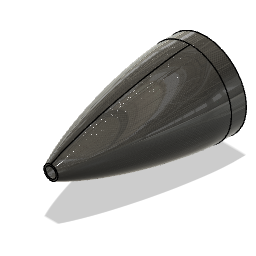
Baugruppe Rakete v7 (Autodesk Fusion 360 archive; units mm, degrees)
design "Nosecone carbon 25.10.2024"
Autodesk Fusion 360 part; units mm, degrees
sketch "Skizze1" plane through (0, 0, 0) normal (1, 0, 0) x (0, 0, -1)
  line L0 (-260, 23.37) -> (-280, 14.04)
  line L1 (-280, 14.04) -> (-290, 8.39)
  line L2 (-260, 23.37) -> (-230, 34.95)
  line L3 (-230, 34.95) -> (-200, 44.83)
  line L4 (-200, 44.83) -> (-160, 56.15)
  line L5 (-160, 56.15) -> (-130, 63.46)
  line L6 (-300, 0) -> (-298, 2.52)
  line L7 (-298, 2.52) -> (-295, 5)
  line L8 (-295, 5) -> (-290, 8.39)
  line L9 (-130, 63.46) -> (-90, 71.77)
  line L10 (-90, 71.77) -> (-40, 79.64)
  line L11 (-40, 79.64) -> (-20, 81.8)
  line L12 (-20, 81.8) -> (0, 83)
  line L13 (0, 83) -> (30, 83)
  line L14 (0, 83) -> (30, 83)
  spline S0 degree 5 poles (0, 83) (-0.9322, 82.957) (-2.773, 82.87) (-5.4634, 82.7359) (-8.9088, 82.5503) (-12.9885, 82.3057) (-16.8689, 82.0449) (-20.6061, 81.7609) (-24.2951, 81.4421) (-28.0746, 81.0712) (-32.1002, 80.6288) (-36.519, 80.0963) (-41.4457, 79.4587) (-46.9344, 78.7077) (-52.9648, 77.8437) (-59.4623, 76.8738) (-66.3117, 75.8102) (-73.373, 74.6692) (-80.4964, 73.4695) (-87.5381, 72.2308) (-94.3743, 70.9725) (-100.9194, 69.7121) (-107.1274, 68.4642) (-112.986, 67.24) (-118.512, 66.0461) (-123.7467, 64.8844) (-128.7513, 63.7504) (-133.602, 62.6333) (-138.3859, 61.5146) (-143.1932, 60.3702) (-148.1077, 59.1751) (-153.1987, 57.9063) (-158.5112, 56.5469) (-164.0583, 55.0892) (-169.8093, 53.5395) (-175.6984, 51.9155) (-181.6391, 50.2416) (-187.5373, 48.5452) (-193.3043, 46.8522) (-198.8707, 45.1828) (-204.1986, 43.5481) (-209.2975, 41.9444) (-214.2149, 40.3564) (-219.0198, 38.7624) (-223.7881, 37.138) (-228.5873, 35.4614) (-233.4626, 33.7172) (-238.4192, 31.9016) (-243.426, 30.0219) (-248.4287, 28.0928) (-253.3595, 26.1341) (-258.1484, 24.1679) (-262.7328, 22.2157) (-267.0706, 20.2957) (-271.1406, 18.4217) (-274.9346, 16.6044) (-278.4519, 14.8519) (-281.6937, 13.1703) (-284.6552, 11.5645) (-287.3272, 10.0386) (-289.706, 8.5968) (-291.8012, 7.243) (-293.6459, 5.983) (-295.2821, 4.8116) (-296.74, 3.695) (-298.0233, 2.5618) (-298.9053, 1.5894) (-299.4846, 0.813) (-299.8343, 0.2745) (-300, 0) knots 0 0 0 0 0 0 0.01538462 0.03076923 0.04615385 0.06153846 0.07692308 0.09230769 0.10769231 0.12307692 0.13846154 0.15384615 0.16923077 0.18461538 0.2 0.21538462 0.23076923 0.24615385 0.26153846 0.27692308 0.29230769 0.30769231 0.32307692 0.33846154 0.35384615 0.36923077 0.38461538 0.4 0.41538462 0.43076923 0.44615385 0.46153846 0.47692308 0.49230769 0.50769231 0.52307692 0.53846154 0.55384615 0.56923077 0.58461538 0.6 0.61538462 0.63076923 0.64615385 0.66153846 0.67692308 0.69230769 0.70769231 0.72307692 0.73846154 0.75384615 0.76923077 0.78461538 0.8 0.81538462 0.83076923 0.84615385 0.86153846 0.87692308 0.89230769 0.90769231 0.92307692 0.93846154 0.95384615 0.96923077 0.98461538 1 1 1 1 1 1
  line L15 (0.1381, 80.0032) -> (30, 80.0032)
  line L16 (30, 80.0032) -> (30, 83)
  spline S1 degree 3 poles (0.1381, 80.0032) (-5.3956, 79.7482) (-10.3945, 79.4727) (-14.9862, 79.1606) (-18.9745, 78.8896) (-22.6391, 78.5928) (-26.579, 78.197) (-30.2006, 77.8332) (-34.1163, 77.3785) (-38.8034, 76.7706) (-43.3782, 76.1772) (-48.6992, 75.4362) (-54.6181, 74.5583) (-62.8597, 73.336) (-72.212, 71.8504) (-81.2998, 70.2728) (-88.6532, 68.9963) (-95.784, 67.6657) (-102.3101, 66.3651) (-109.346, 64.9629) (-115.6909, 63.5997) (-121.531, 62.2994) (-130.6599, 60.2669) (-138.6135, 58.4165) (-147.4068, 56.2505) (-152.4678, 55.0039) (-157.8323, 53.634) (-163.547, 52.1114) (-171.5204, 49.9869) (-180.1377, 47.5749) (-188.3041, 45.1883) (-193.9882, 43.5271) (-199.4138, 41.8911) (-204.4798, 40.3083) (-210.9231, 38.295) (-216.8267, 36.3556) (-222.7977, 34.2958) (-227.6528, 32.6209) (-232.5948, 30.8535) (-237.6449, 28.9777) (-245.8863, 25.9164) (-254.3169, 22.5835) (-261.6486, 19.3972) (-270.0166, 15.7604) (-276.9857, 12.3321) (-282.3719, 9.3784) (-285.7999, 7.4985) (-288.5366, 5.8129) (-290.7419, 4.3239) (-292.7166, 2.9906) (-294.3202, 1.8334) (-295.4633, 0.7925) (-296.31, 0.0214) (-296.9311, -0.7211) (-297.4317, -1.5504) knots 0 0 0 0 0.054964 0.054964 0.054964 0.102705 0.102705 0.102705 0.14659 0.14659 0.14659 0.189423 0.189423 0.189423 0.249066 0.249066 0.249066 0.297325 0.297325 0.297325 0.349355 0.349355 0.349355 0.430685 0.430685 0.430685 0.477496 0.477496 0.477496 0.542809 0.542809 0.542809 0.58827 0.58827 0.58827 0.646091 0.646091 0.646091 0.693105 0.693105 0.693105 0.769829 0.769829 0.769829 0.857397 0.857397 0.857397 0.91313 0.91313 0.91313 0.963033 0.963033 0.963033 1 1 1 1
  line L17 (-300, 0) -> (-296.2633, 0)
  line L18 (-280, 14.04) -> (-280, 10.6551)
  dimension "d1" = 10
  dimension "d2" = 8.39
  dimension "d4" = 20
  dimension "d5" = 40
  dimension "d6" = 70
  dimension "d7" = 300
  dimension "d8" = 100
  dimension "d9" = 140
  dimension "d10" = 170
  dimension "d11" = 14.04
  dimension "d12" = 2
  dimension "d13" = 5
  dimension "d14" = 2.52
  dimension "d15" = 5
  dimension "d16" = 23.37
  dimension "d17" = 34.95
  dimension "d18" = 44.83
  dimension "d19" = 56.15
  dimension "d20" = 63.46
  dimension "d21" = 210
  dimension "d22" = 260
  dimension "d23" = 71.77
  dimension "d24" = 79.64
  dimension "d25" = 83
  dimension "d26" = 280
  dimension "d27" = 81.8
  dimension "d28" = 30
  dimension "d30" = -3
  constraint horizontal origin L6.start
  constraint vertical origin L12.end
  constraint horizontal L13
  constraint parallel L14 L15
  constraint vertical L16
  constraint coincident L15.start S1.start
  constraint coincident S1 L17.end
  constraint horizontal L17
  constraint coincident L0.end L1.start
  constraint coincident S1 L18.end
  constraint vertical L18
  measures "d1" horizontal distance of L1.end L6.start
  measures "d2" vertical distance of L1.end L6.start
  measures "d4" horizontal distance of L0.end L6.start
  measures "d5" horizontal distance of L0.start L6.start
  measures "d6" horizontal distance of L6.start L2.end
  measures "d7" distance of origin L6.start
  measures "d8" horizontal distance of L3.end L6.start
  measures "d9" horizontal distance of L6.start L4.end
  measures "d10" horizontal distance of L6.start L5.end
  measures "d11" vertical distance of L0.end L6.start
  measures "d12" horizontal distance of L6.start L6.end
  measures "d13" horizontal distance of L6.start L7.end
  measures "d14" vertical distance of L6.start L6.end
  measures "d15" vertical distance of L6.start L7.end
  measures "d16" vertical distance of L0.start L6.start
  measures "d17" vertical distance of L6.start L2.end
  measures "d18" vertical distance of L3.end L6.start
  measures "d19" vertical distance of L6.start L4.end
  measures "d20" vertical distance of L6.start L5.end
  measures "d21" horizontal distance of L6.start L9.end
  measures "d22" horizontal distance of L6.start L10.end
  measures "d23" vertical distance of L6.start L9.end
  measures "d24" vertical distance of L6.start L10.end
  measures "d25" vertical distance of L6.start L12.end
  measures "d26" horizontal distance of L6.start L11.end
  measures "d27" vertical distance of L6.start L11.end
  measures "d28" distance of L12.end L13.end
revolve "Drehen1" add sketch "Skizze1" angle 360 about axis through (0, 0, 1.75) along (0, 0, 1) contours L0 L2 L3 L4 L5 L9 L10 L11 L12 L13 L14 L15 L16 S1 L18 | L2 S0 | L0 S0 | L3 S0 | L4 S0 | L5 S0 | L9 S0 | L10 S0 | L12 S0 | L11 S0
fillet "Abrundung1" radius 2 1 edges at (-74.5892, 28.9304, -30)

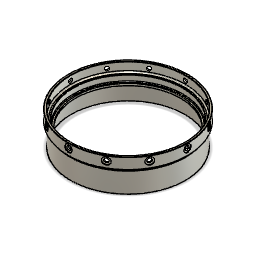
design "Connection-Ring-female-21.10.2024"
Autodesk Fusion 360 part; units mm, degrees
sketch "Skizze1" plane through (0, 0, 0) normal (0, 0, 1) x (1, 0, 0)
  line L0 (-83, 47) -> (-83, 30)
  line L1 (-83, 30) -> (-80, 30)
  line L2 (-80, 30) -> (-80, 0)
  line L3 (-73, 22.5) -> (-73, 25.5)
  line L4 (-73, 25.5) -> (-76, 25.5)
  line L5 (-76, 25.5) -> (-76, 34)
  line L6 (-76, 34) -> (-80, 34)
  line L7 (-80, 34) -> (-80, 47)
  line L8 (-80, 47) -> (-83, 47)
  line L9 (-80, 0) -> (-79, 0)
  line L10 (-76.75, 22.5) -> (-73, 22.5)
  line L11 (-76.75, 22.5) -> (-79, 0)
  line L12 (-76, 30) -> (-76.75, 22.5)
  dimension "d2" = 3
  dimension "d6" = 13
  dimension "d7" = 80
  dimension "d8" = 3
  dimension "d9" = 4
  dimension "d10" = 3
  dimension "d21" = 4
  dimension "d22" = 8.5
  dimension "d23" = 3
  dimension "d24" = 30
  dimension "d25" = 1
  constraint vertical L0
  constraint perpendicular L0 L1
  constraint perpendicular L1 L2
  constraint perpendicular L2 L4
  constraint perpendicular L5 L6
  constraint perpendicular L6 L7
  constraint perpendicular L0 L8
  constraint perpendicular L2 L9
  constraint horizontal origin L2.end
  constraint coincident L5 L12.start
  constraint collinear L11 L12
  constraint horizontal L1.end L12.start
  measures "d2" distance of L3 L5
  measures "d6" distance of L6 L8
  measures "d7" distance of origin L2
  measures "d8" distance of L0 L7
  measures "d9" distance of L2 L5
  measures "d10" distance of L0 L2
  measures "d21" distance of L1 L6
  measures "d22" distance of L4 L6
  measures "d23" distance of L4 L10
  measures "d24" distance of L1 L9
  measures "d25" distance of L2.end L9.end
revolve "Drehen1" add sketch "Skizze1" angle 360 about axis through (0, 1.75, 0) along (0, 1, 0)
fillet "Abrundung1" radius 2 1 edges at (-77.3832, 30, 30.0141)
fillet "Abrundung2" radius 2 1 edges at (-74.5862, 30, 28.9292)
fillet "Abrundung3" radius 2 1 edges at (-74.5862, 34, 28.9292)
chamfer "Fase3" distance 1 angle 45 1 edges at (-70.8569, 25.5, 27.4828)
ref_plane "Arbeitsebene1" through (83, 38.5, 0) normal (1, 0, 0) x (0, 0, -1)
sketch "Skizze4" plane through (83, 0, 0) normal (1, 0, 0) x (0, 0, -1)
  line L0 (-82.5, 47) -> (82.5, 47)
  point P0 (0, 40.5)
  dimension "d34" = 6.5
  constraint vertical origin P0
  measures "d34" distance of P0 L0
hole "Bohrung2" at (83, 40.5, 0) direction (-1, 0, 0) diameter 5.5 depth 16 tip angle 118 counterbore diameter 10 counterbore depth 1
pattern_circular "C-Anordnung1" count 12 over 360 about axis through (0, 1.75, 0) along (0, 1, 0) of "Bohrung2"
chamfer "Fase4" distance 0.4 angle 45 7 edges at (-74.5862, 47, 28.9292) (-70.8569, 34, 27.4828) (-74.5862, 0, 28.9292) (-73.6539, 0, 28.5676) (-71.5561, 22.5, 27.754) (-68.0599, 22.5, 26.3979) (-77.3832, 47, 30.0141)
equation "d7 = ( 160 / 2 ) * 1 mm"
equation "d22 = 15 mm - d6 / 2"

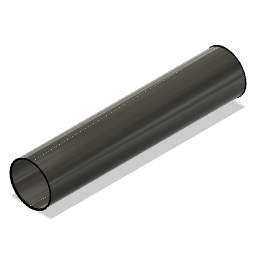
design "Computer/Nutzlastsektion 800"
Autodesk Fusion 360 part; units mm, degrees
sketch "Skizze1" plane through (0, 0, 0) normal (0, 0, 1) x (1, 0, 0)
  circle A0 centre (0, 0) radius 80
  circle A1 centre (0, 0) radius 83
  dimension "d1" = 166
  dimension "d2" = 160
  constraint coincident A0.centre A1.centre
  constraint concentric A0 A1
  measures "d1" diameter of A1
  measures "d2" diameter of A0
extrude "Extrusion1" add sketch "Skizze1" along normal blind 800
fillet "Abrundung1" radius 2 2 edges at (-74.5862, 28.9292, 800) (-74.5862, 28.9292, 0)

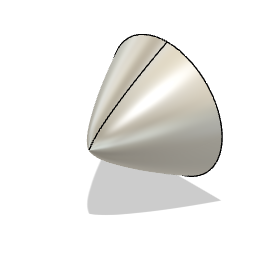
design "Nasenspitze"
Autodesk Fusion 360 part; units mm, degrees
sketch "Skizze1" plane through (0, 0, 0) normal (1, 0, 0) x (0, 0, -1)
  line L0 (-18, 2.52) -> (-15, 5)
  line L1 (-15, 5) -> (-10, 8.39)
  line L2 (0, 14.04) -> (-10, 8.39)
  line L3 (-20, 0) -> (-18, 2.52)
  spline S0 degree 5 poles (0, 14.04) (-0.347, 13.8595) (-1.0331, 13.5009) (-2.0382, 12.9697) (-3.3302, 12.2751) (-4.8637, 11.4299) (-6.3143, 10.6085) (-7.6808, 9.8116) (-8.9624, 9.0402) (-10.1599, 8.2952) (-11.2757, 7.5774) (-12.3148, 6.8876) (-13.2837, 6.2257) (-14.189, 5.5902) (-15.0369, 4.9781) (-15.8322, 4.3839) (-16.5772, 3.7988) (-17.2729, 3.2129) (-17.9192, 2.6164) (-18.5158, 2.001) (-19.0631, 1.362) (-19.4619, 0.8303) (-19.7393, 0.4197) (-19.9147, 0.1408) (-20, 0) knots 0 0 0 0 0 0 0.05 0.1 0.15 0.2 0.25 0.3 0.35 0.4 0.45 0.5 0.55 0.6 0.65 0.7 0.75 0.8 0.85 0.9 0.95 1 1 1 1 1 1
  line L4 (-20, 0) -> (-15, 0)
  line L5 (0, 10) -> (0, 14.04)
  line L6 (0, 10) -> (-14.017, 1.7221)
  arc A0 (-14.017, 1.7221) -> (-15, 0) centre (-13, 0) ccw
  point P0 (-297.4317, -1.5504)
  dimension "d1" = 10
  dimension "d2" = 8.39
  dimension "d3" = 20
  dimension "d4" = 14.04
  dimension "d5" = 2
  dimension "d6" = 5
  dimension "d7" = 2.52
  dimension "d8" = 5
  dimension "d9" = 15
  dimension "d10" = 10
  dimension "d11" = 2
  constraint vertical origin L2.start
  constraint horizontal origin L3.start
  constraint horizontal L4
  constraint vertical L5
  constraint tangent L6 A0
  constraint horizontal origin A0.centre
  measures "d1" horizontal distance of L3.start L1.end
  measures "d2" vertical distance of L3.start L1.end
  measures "d3" horizontal distance of L3.start L2.start
  measures "d4" vertical distance of L3.start L2.start
  measures "d5" horizontal distance of L3.start L0.start
  measures "d6" horizontal distance of L3.start L0.end
  measures "d7" vertical distance of L3.start L0.start
  measures "d8" vertical distance of L3.start L0.end
  measures "d9" distance of origin L4.end
  measures "d10" distance of origin L5.start
  measures "d11" radius of A0
revolve "Drehen1" add sketch "Skizze1" angle 360 about axis through (0, 0, 1.75) along (0, 0, 1)

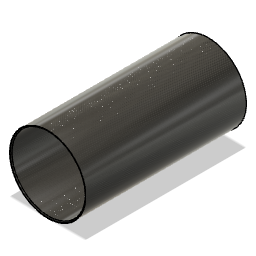
design "Antriebssektion 2 350"
Autodesk Fusion 360 part; units mm, degrees
sketch "Skizze1" plane through (0, 0, 0) normal (0, 0, 1) x (1, 0, 0)
  circle A0 centre (0, 0) radius 83
  circle A1 centre (0, 0) radius 80
  dimension "d1" = 160
  dimension "d2" = 166
  constraint coincident A0.centre A1.centre
  measures "d1" diameter of A1
  measures "d2" diameter of A0
extrude "Extrusion1" add sketch "Skizze1" along normal blind 350
fillet "Abrundung1" radius 2 2 edges at (-74.5862, 28.9292, 350) (-74.5862, 28.9292, 0)

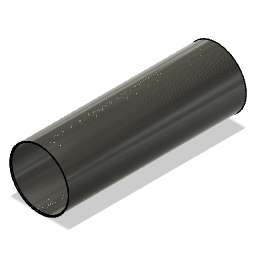
design "Antriebssektion 1 500"
Autodesk Fusion 360 part; units mm, degrees
sketch "Skizze1" plane through (0, 0, 0) normal (0, 0, 1) x (1, 0, 0)
  circle A0 centre (0, 0) radius 83
  circle A1 centre (0, 0) radius 80
  dimension "d1" = 166
  dimension "d2" = 160
  constraint coincident A0.centre A1.centre
  constraint concentric A0 A1
  measures "d1" diameter of A0
  measures "d2" diameter of A1
extrude "Extrusion1" add sketch "Skizze1" along normal blind 500
fillet "Abrundung1" radius 2 2 edges at (-74.5862, 28.9292, 500) (-74.5862, 28.9292, 0)

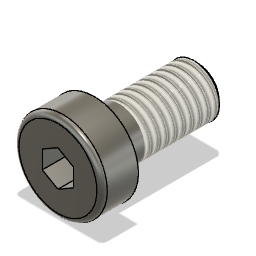
design "Innensechskantschraube DIN 7984 - M5 x 10 Stahl 8.8 Einfach"
description: Innensechskantschraube DIN 7984 - M5 x 10
Autodesk Fusion 360 part; units mm, degrees
sketch "Sketch1" plane through (0, 0, 0) normal (0, 1, 0) x (1, 0, 0)
  line L0 (-2.5, 0) -> (-2.5, 10)
  line L1 (-2.5, 10) -> (0, 10)
  line L2 (0, 10) -> (0, -3.5)
  line L3 (-2.5, 0) -> (-4.25, 0)
  line L4 (-4.25, 0) -> (-4.25, -3.5)
  line L5 (-4.25, -3.5) -> (0, -3.5)
  dimension "d9" = 5
  dimension "d66" = 8.5
  dimension "d68" = 10
  dimension "d79" = 3.5
  constraint perpendicular L0 L1
  constraint collinear origin L1.end L2.end
  constraint perpendicular L0 L3
  constraint coincident origin L3
  constraint vertical L0
  constraint vertical L2
  constraint parallel L2 L4
  constraint coincident L2 L5.end
  constraint perpendicular L2 L5
  measures "d68" distance of origin L1.end
  measures "d79" distance of L3.end L4.end
revolve "Revolve1" add sketch "Sketch1" angle 360 about axis through (0, 0, -10) along (0, 0, 1)
ref_plane "WorkPlane1" through (0, 0, 3.5) normal (0, 0, 1) x (1, 0, 0)
sketch "Sketch6" plane through (0, 0, 3.5) normal (0, 0, 1) x (1, 0, 0)
  line L0 (-1.5, 0) -> (1.5, 0) construction
  line L1 (0, 0) -> (-1.5, 0.866)
  line L2 (-1.5, -0.866) -> (-1.5, 0.866)
  line L3 (-1.5, -0.866) -> (0, 0)
  dimension "d72" = 3
  dimension "d100" = 150
  constraint horizontal L0
  constraint midpoint L1.start L0
  constraint coincident L1.start L3.end
  constraint perpendicular L0 L2
  constraint midpoint L0.start L2
  constraint coincident L1.end L2.end
  measures "d72" distance of L0.start L0.end
  measures "d100" angle of L0 L1
extrude "Extrude1" cut sketch "Sketch6" against normal blind 2.7
pattern_circular "C-Pattern1" count 6 over 360 about axis through (0, 0, 1.75) along (0, 0, 1) of "Extrude1"
extrude "Extrude2" cut 1 faces at (0, -0.5774, 0.8) along direction (0, 0, -1) blind 2.7 draft -85
thread "Thread2" "ISO Metric profile 5.0 M5x0.8 6g" major diameter 4.901 minor diameter 3.9895 pitch 0.8 angle 60 resizes the face on face at (-2.4876, 0.2489, -3.3333) from (0, 0, -2.4) to (0, 0, -10)
fillet "Fillet4" radius 0.5 1 edges at (-3.9624, 1.5369, 3.5)
sketch "Sketch7" plane through (0, 0, 0) normal (0, 1, 0) x (1, 0, 0)
  line L0 (-2.55, 10) -> (-2.55, 9.5092)
  line L1 (-2.55, 9.5092) -> (-2.0092, 10)
  line L2 (0, 10) -> (0, -3.5)
  line L3 (-2.55, 10) -> (0, 10)
  dimension "d92" = 0.4908
  dimension "d98" = 2.0092
  dimension "d99" = 2.55
  constraint coincident L2.start L3.end
  constraint perpendicular L2 L3
  constraint coincident L1.end L3
  constraint perpendicular L0 L3
  measures "d92" vertical distance of L0.end L1.end
  measures "d98" horizontal distance of origin L1.end
  measures "d99" distance of origin L0
revolve "Revolve3" cut sketch "Sketch7" angle 360 about axis through (0, 0, 1.75) along (0, 0, 1)
equation "d9 = adsk_nomdia"
equation "adsk_nomlen = 10.00 mm"
equation "adsk_headh = 3.50 mm"
equation "adsk_headdia = 8.50 mm"
equation "adsk_nomdia = 5.00 mm"
equation "adsk_philwidth = 3.00 mm"
equation "d31 = -adsk_phildepth"
equation "adsk_phildepth = 2.70 mm"
equation "d66 = adsk_headdia"
equation "d68 = adsk_nomlen"
equation "d71 = adsk_headh"
equation "d72 = adsk_philwidth"
equation "d76 = -adsk_phildepth"
equation "d79 = adsk_headh"
equation "adsk_thrlen = 7.60 mm"
equation "d84 = adsk_thrlen"
equation "d86 = adsk_nomdia * 0.1"
equation "d92 = adsk_startlen"
equation "adsk_startlen = 0.49076 mm"
equation "adsk_endpointdia = 4.01848 mm"
equation "d98 = adsk_endpointdia / 2"
equation "d99 = adsk_nomdia * 0.51"

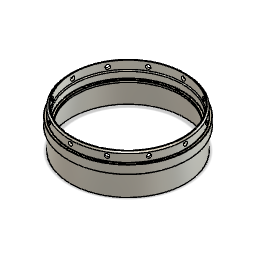
design "Connection-Ring-male-21.10.2024"
Autodesk Fusion 360 part; units mm, degrees
sketch "Skizze1" plane through (0, 0, 0) normal (0, 0, 1) x (1, 0, 0)
  line L0 (-80, 0) -> (-80, 30)
  line L1 (-80, 30) -> (-83, 30)
  line L2 (-83, 30) -> (-83, 42)
  line L3 (-83, 42) -> (-79.95, 42)
  line L4 (-79.95, 42) -> (-79.95, 53)
  line L5 (-77.95, 55) -> (-76.95, 55)
  line L6 (-76.95, 55) -> (-76.95, 42)
  line L7 (-76, 33.5) -> (-73, 33.5)
  line L8 (-73, 30.5) -> (-73, 33.5)
  line L9 (-77.95, 55) -> (-79.95, 53)
  line L10 (-80, 0) -> (-79, 0)
  line L11 (-73, 30.5) -> (-75.95, 30.5)
  line L12 (-75.95, 30.5) -> (-79, 0)
  line L13 (-76, 30) -> (-75.95, 30.5)
  line L14 (-76.95, 42) -> (-76, 42)
  line L15 (-76, 42) -> (-76, 33.5)
  dimension "d1" = 3
  dimension "d2" = 80
  dimension "d5" = 3
  dimension "d7" = 3.05
  dimension "d9" = 2
  dimension "d10" = 3
  dimension "d13" = 1
  dimension "d14" = 30
  dimension "d16" = 2
  dimension "d17" = 4
  dimension "d18" = 8.5
  dimension "d19" = 13
  dimension "d20" = 12
  dimension "d25" = 3
  constraint perpendicular L0 L1
  constraint perpendicular L1 L2
  constraint perpendicular L2 L3
  constraint perpendicular L3 L4
  constraint perpendicular L4 L5
  constraint perpendicular L3 L6
  constraint perpendicular L4 L7
  constraint perpendicular L7 L8
  constraint perpendicular L0 L10
  constraint vertical L8
  constraint perpendicular L8 L11
  constraint horizontal origin L0.start
  constraint collinear L12 L13
  constraint horizontal L0.end L13.start
  constraint perpendicular L6 L14
  constraint perpendicular L14 L15
  constraint vertical L7.start L13.start
  constraint collinear L3 L14
  measures "d1" distance of L7.end L8.start
  measures "d2" distance of origin L0
  measures "d5" distance of L4 L6
  measures "d7" distance of L2 L4
  measures "d9" distance of L4 L5.start
  measures "d10" distance of L0 L2
  measures "d13" distance of L0.start L10.end
  measures "d14" distance of L1 L10
  measures "d16" distance of L5 L4.end
  measures "d17" distance of L0.end L13.start
  measures "d18" distance of L3 L7
  measures "d19" distance of L3 L5
  measures "d20" distance of L1 L3
  measures "d25" distance of L8 L15
revolve "Drehen1" add sketch "Skizze1" angle 360 about axis through (0, 1.75, 0) along (0, 1, 0)
fillet "Abrundung1" radius 2 1 edges at (-71.7426, 42, 27.8263)
ref_plane "Arbeitsebene1" through (79.95, 47.5, 0) normal (1, 0, 0) x (0, 0, -1)
sketch "Skizze2" plane through (79.95, 0, 0) normal (1, 0, 0) x (0, 0, -1)
  line L0 (77.95, 55) -> (-77.95, 55)
  point P0 (0, 48.5)
  dimension "d27" = 6.5
  constraint vertical origin P0
  measures "d27" distance of P0 L0
hole "Bohrung1" at (79.95, 48.5, 0) direction (-1, 0, 0) diameter 5.5 depth 16 tip angle 118
pattern_circular "C-Anordnung1" count 12 over 360 about axis through (0, 1.75, 0) along (0, 1, 0) of "Bohrung1"
chamfer "Fase1" distance 0.4 angle 45 9 edges at (-77.3832, 42, 30.0141) (-77.3832, 30, 30.0141) (-73.6539, 0, 28.5676) (-70.8103, 30.5, 27.4647) (-68.0599, 30.5, 26.3979) (-70.8569, 33.5, 27.4828) (-74.5396, 42, 28.9112) (-74.5862, 0, 28.9292) (-68.0599, 33.5, 26.3979)
fillet "Abrundung2" radius 2 1 edges at (-74.5862, 30, 28.9292)
equation "d2 = ( 160 / 2 ) * 1 mm"
equation "d18 = 15 mm - d19 / 2"

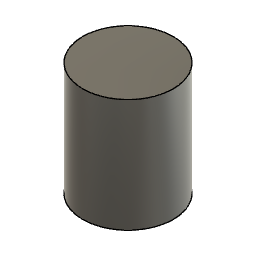
design "Bolzen"
Autodesk Fusion 360 part; units mm, degrees
sketch "Skizze1" plane through (0, 0, 0) normal (0, 1, 0) x (1, 0, 0)
  circle A0 centre (0, 0) radius 2
  dimension "d1" = 4
  constraint coincident A0.centre origin
  measures "d1" diameter of A0
extrude "Extrusion1" add sketch "Skizze1" along normal blind 5

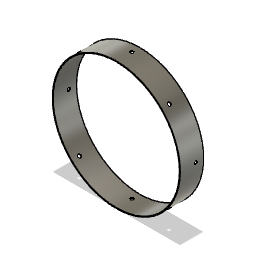
design "Kupplungsring Verbinder 25.10.2024"
Autodesk Fusion 360 part; units mm, degrees
sketch "Skizze2" plane through (0, 0, 0) normal (0, 0, 1) x (1, 0, 0)
  circle A0 centre (0, 0) radius 82
  circle A1 centre (0, 0) radius 81
  dimension "d1" = 164
  dimension "d2" = 162
  constraint coincident A0.centre A1.centre
  constraint concentric A0 A1
  measures "d1" diameter of A0
  measures "d2" diameter of A1
extrude "Extrusion1" add sketch "Skizze2" along normal blind 30
ref_plane "Arbeitsebene1" through (0, 82, 15) normal (0, 1, 0) x (-1, 0, 0)
sketch "Skizze3" plane through (0, 82, 0) normal (0, 1, 0) x (1, 0, 0)
  point P0 (0, -10)
  dimension "d6" = 10
  constraint vertical origin P0
  measures "d6" distance of origin P0
ref_plane "Arbeitsebene2" through (-57.9828, 57.9828, 15) normal (-0.707107, 0.707107, 0) x (-0.707107, -0.707107, 0)
sketch "Skizze4" plane through (-57.9828, 57.9828, 0) normal (-0.707107, 0.707107, 0) x (-0.707107, -0.707107, 0)
  line L0 (82, 30) -> (-82, 30)
  point P0 (0, 20)
  dimension "d8" = 10
  constraint vertical origin P0
  measures "d8" distance of P0 L0
hole "Bohrung1" at (0, 82, 10) direction (0, -1, 0) diameter 4 depth 35 tip angle 118
hole "Bohrung2" at (-57.9828, 57.9828, 20) direction (0.707107, -0.707107, 0) diameter 4 depth 35 tip angle 118
pattern_circular "C-Anordnung1" count 4 over 360 about axis through (0, 0, 1.75) along (0, 0, 1) of "Bohrung1", "Bohrung2"

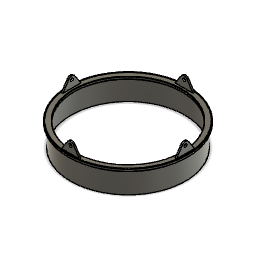
design "Kupplungsring 25.10.2024"
Autodesk Fusion 360 part; units mm, degrees
sketch "Skizze1" plane through (0, 0, 0) normal (0, 0, 1) x (1, 0, 0)
  line L0 (-80, 0) -> (-79, 0)
  line L1 (-79, 0) -> (-77, 30)
  line L2 (-77, 30) -> (-75, 30)
  line L3 (-75, 30) -> (-75, 33)
  line L4 (-80, 30) -> (-80, 0)
  line L5 (-80, 30) -> (-83, 30)
  line L6 (-83, 30) -> (-83, 35)
  line L7 (-82, 33) -> (-75, 33)
  line L8 (-83, 35) -> (-83, 33.5)
  line L9 (-83, 33.5) -> (-82, 33.5)
  line L10 (-82, 33.5) -> (-82, 33)
  dimension "d1" = 80
  dimension "d2" = 1
  dimension "d3" = 3
  dimension "d4" = 30
  dimension "d5" = 8
  dimension "d6" = 3
  dimension "d7" = 3
  dimension "d8" = 1
  dimension "d9" = 0.5
  constraint horizontal L0
  constraint parallel L0 L2
  constraint perpendicular L2 L3
  constraint perpendicular L0 L4
  constraint horizontal origin L0.end
  constraint perpendicular L4 L5
  constraint perpendicular L5 L6
  constraint horizontal L7
  constraint horizontal L1.end L4.start
  constraint perpendicular L7 L8
  constraint perpendicular L8 L9
  constraint perpendicular L7 L10
  measures "d1" distance of origin L0.start
  measures "d2" distance of L0.start L0.end
  measures "d3" distance of L1.end L4
  measures "d4" distance of L0 L5
  measures "d5" distance of L2.end L5.end
  measures "d6" distance of L4.start L5.end
  measures "d7" distance of L5 L7
  measures "d8" distance of L8 L10
  measures "d9" distance of L7 L9
revolve "Drehen1" add sketch "Skizze1" angle 360 about axis through (0, 1.75, 0) along (0, 1, 0)
fillet "Abrundung1" radius 2 2 edges at (-74.5862, 30, 28.9292) (-71.7892, 30, 27.8444)
chamfer "Fase1" distance 0.5 angle 45 3 edges at (-77.3832, 30, 30.0141) (-77.3832, 33.5, 30.0141) (-69.9246, 33, 27.1212)
sketch "Skizze2" plane through (0, 0, 0) normal (0, 0, 1) x (1, 0, 0)
  line L0 (82, 33) -> (-82, 33)
  line L1 (75.5, 33) -> (-75.5, 33)
  line L2 (-82.5, 33.5) -> (82.5, 33.5)
  arc A0 (4.1867, 45.7334) -> (-4.1867, 45.7334) centre (0, 43) ccw
  line L3 (-4.1867, 45.7334) -> (-12.5, 33)
  line L4 (4.1867, 45.7334) -> (12.5, 33)
  circle A1 centre (0, 43) radius 2
  dimension "d14" = 5
  dimension "d16" = 10
  dimension "d17" = 25
  dimension "d18" = 4
  constraint vertical origin A0.centre
  constraint coincident L1 L3.end
  constraint coincident L1 L4.end
  constraint tangent A0 L3
  constraint tangent A0 L4
  constraint equal L3 L4
  constraint concentric A0 A1
  measures "d14" radius of A0
  measures "d16" distance of L0 A0.centre
  measures "d17" distance of L3.end L4.end
  measures "d18" diameter of A1
ref_plane "Arbeitsebene1" through (0, 33.25, -82) normal (0, 0, -1) x (-1, 0, 0)
extrude "Extrusion1" add sketch "Skizze2" along normal blind 2 from surface at -80
pattern_circular "C-Anordnung1" count 4 over 360 about axis through (0, 1.75, 0) along (0, 1, 0) of "Extrusion1"
equation "d1 = ( 160 / 2 ) * 1 mm"

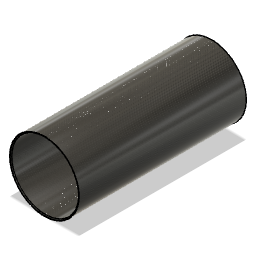
design "Fallschirmsektion 1,2 400"
Autodesk Fusion 360 part; units mm, degrees
sketch "Skizze1" plane through (0, 0, 0) normal (0, 0, 1) x (1, 0, 0)
  circle A0 centre (0, 0) radius 80
  circle A1 centre (0, 0) radius 83
  dimension "d1" = 160
  dimension "d2" = 166
  constraint coincident A0.centre A1.centre
  measures "d1" diameter of A0
  measures "d2" diameter of A1
extrude "Extrusion1" add sketch "Skizze1" along normal blind 400
fillet "Abrundung1" radius 2 2 edges at (-74.5862, 28.9292, 400) (-74.5862, 28.9292, 0)
